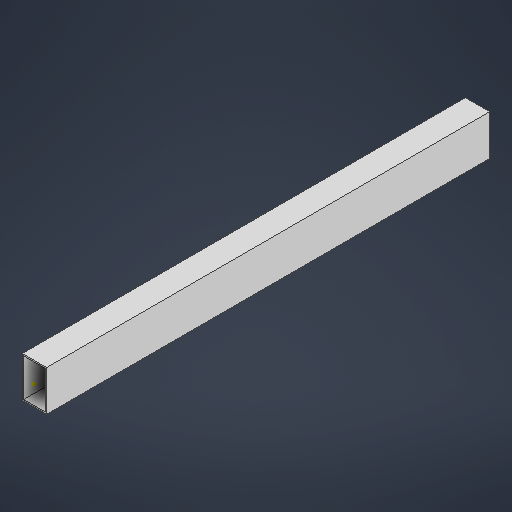
# Autodesk Inventor part: 321x30
Saved by Autodesk Inventor 2025 (Build 290162000, 162)
## iProperties
Created: 2025-11-08
Part Number: 321x30
Material: 常规
Document SubType Name: Modeling
Designer: XH
Density: 1 g/cm^3
Appearance: 默认
Author: XH
Autodesk Inventor part; units mm, degrees
ref_plane "YZ Plane" through (0, 0, 0) normal (1, 0, 0) x (0, 1, 0)
ref_plane "XZ Plane" through (0, 0, 0) normal (0, 1, 0) x (-1, 0, 0)
ref_plane "XY Plane" through (0, 0, 0) normal (0, 0, 1) x (1, 0, 0)
sketch "草图1" plane through (0, 0, 0) normal (0, 0, 1) x (1, 0, 0)
  line L0 (9, -15) -> (-9, -15)
  line L1 (-9, -15) -> (-9, 15)
  line L2 (-9, 15) -> (9, 15)
  line L3 (9, 15) -> (9, -15)
  line L4 (9, -15) -> (-9, 15) construction
  line L5 (-9, -15) -> (9, 15) construction
  line L6 (8, 14) -> (-8, 14)
  line L7 (-8, 14) -> (-8, -14)
  line L8 (-8, -14) -> (8, -14)
  line L9 (8, -14) -> (8, 14)
  point P0 (0, 0)
  dimension "d0" = 30
  dimension "d1" = 18
  dimension "d4" = 1
  constraints: 20 end point, 4 parallel, 2 midpoint, 2 perpendicular, 1 horizontal, 3 other
  measures "d0" distance of L0.end L1.end
  measures "d1" distance of L0.start L0.end
  measures "d4" distance between parallel lines of L2 L6
extrude "拉伸1" add sketch "草图1" along normal blind 328
sketch "草图2" plane through (0, 0, 328) normal (0, 0, 1) x (1, 0, 0)
  point P0 (0, 0)
